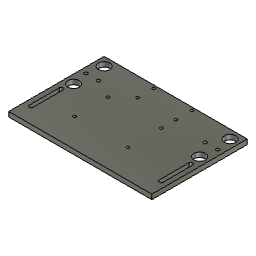
RollerPlate v14 (Autodesk Fusion 360 design; units mm, degrees)
Autodesk Fusion 360 part; units mm, degrees
sketch "Sketch1" plane through (0, 0, 0) normal (0, 0, 1) x (1, 0, 0)
  line L0 (-150, 100) -> (0, 100)
  line L1 (0, 100) -> (0, 0)
  line L2 (0, 0) -> (-150, 0)
  line L3 (-150, 0) -> (-150, 100)
  circle A0 centre (-135, 75) radius 3.25
  circle A1 centre (-115, 75) radius 3.25
  circle A2 centre (-35, 75) radius 3.25
  circle A3 centre (-15, 75) radius 3.25
  line L4 (-141, 48) -> (-141, 22)
  line L5 (-145, 22) -> (-145, 48)
  arc A4 (-143, 50) -> (-145, 48) centre (-143, 48) ccw
  arc A5 (-141, 48) -> (-143, 50) centre (-143, 48) ccw
  arc A6 (-145, 22) -> (-143, 20) centre (-143, 22) ccw
  arc A7 (-143, 20) -> (-141, 22) centre (-143, 22) ccw
  line L6 (-5, 48) -> (-5, 22)
  line L7 (-9, 22) -> (-9, 48)
  arc A8 (-7, 50) -> (-9, 48) centre (-7, 48) ccw
  arc A9 (-5, 48) -> (-7, 50) centre (-7, 48) ccw
  arc A10 (-9, 22) -> (-7, 20) centre (-7, 22) ccw
  arc A11 (-7, 20) -> (-5, 22) centre (-7, 22) ccw
  point P0 (-145, 50)
  point P1 (-141, 50)
  point P2 (-9, 50)
  point P3 (-5, 50)
  dimension "d1" = 150
  dimension "d2" = 100
  dimension "d3" = 6.5
  dimension "d4" = 25
  dimension "d5" = 15
  dimension "d6" = 6.5
  dimension "d7" = 6.5
  dimension "d8" = 6.5
  dimension "d9" = 20
  dimension "d10" = 15
  dimension "d11" = 20
  dimension "d53" = 4
  dimension "d55" = 5
  dimension "d57" = 2
  dimension "d58" = 2
  dimension "d59" = 2
  dimension "d60" = 4
  dimension "d62" = 5
  dimension "d64" = 2
  dimension "d65" = 2
  dimension "d66" = 2
  dimension "d67" = 2
  constraint horizontal L0
  constraint vertical L1
  constraint horizontal L2
  constraint vertical L3
  constraint coincident L1.end L2.start
  constraint vertical L4
  constraint vertical L5
  constraint coincident P0 L5
  constraint tangent L5 A4
  constraint coincident P1 L4
  constraint tangent L4 A5
  constraint coincident A4.start A5.end
  constraint tangent L5 A6
  constraint tangent L4 A7
  constraint equal A6 A7
  constraint coincident A6.end A7.start
  constraint vertical L6
  constraint vertical L7
  constraint coincident P2 L7
  constraint tangent L7 A8
  constraint coincident P3 L6
  constraint tangent L6 A9
  constraint coincident A8.start A9.end
  constraint tangent L7 A10
  constraint tangent L6 A11
  constraint coincident A10.end A11.start
  measures "d1" distance of L1 L3
  measures "d2" distance of L0 L2
  measures "d3" diameter of A0
  measures "d4" distance of L0 A0.centre
  measures "d5" distance of L3 A0.centre
  measures "d6" diameter of A1
  measures "d7" diameter of A2
  measures "d8" diameter of A3
  measures "d9" distance of A0.centre A1.centre
  measures "d10" distance of L1 A3.centre
  measures "d11" distance of A2.centre A3.centre
  measures "d53" distance of P0 P1
  measures "d55" distance of L3 L5
  measures "d57" radius of A4
  measures "d58" radius of A5
  measures "d59" radius of A6
  measures "d60" distance of P2 P3
  measures "d62" distance of L1 L6
  measures "d64" radius of A8
  measures "d65" radius of A9
  measures "d66" radius of A10
  measures "d67" radius of A11
extrude "Extrude1" add sketch "Sketch1" along normal blind 5 contours L0 L1 L2 L3 | L4 L5 A4 A5 A6 A7 | L6 L7 A8 A9 A10 A11 makes body 1
sketch "Sketch2" plane through (0, 0, 5) normal (0, 0, 1) x (-1, 0, 0)
  circle A0 centre (135, -75) radius 3.25
  circle A1 centre (35, -75) radius 3.25
  circle A2 centre (115, -75) radius 3.25
  circle A3 centre (15, -75) radius 3.25
  line L0 (150, 0) -> (0, 0)
  line L1 (0, 0) -> (0, -100)
  line L2 (0, -100) -> (150, -100)
  line L3 (150, -100) -> (150, 0)
  circle A4 centre (141, -91) radius 6
  circle A5 centre (141, -59) radius 6
  circle A6 centre (109, -91) radius 6
  circle A7 centre (109, -59) radius 6
  circle A8 centre (41, -91) radius 6
  circle A9 centre (41, -59) radius 6
  circle A10 centre (9, -91) radius 6
  circle A11 centre (9, -59) radius 6
  dimension "d25" = 12
  dimension "d26" = 9
  dimension "d27" = 9
  dimension "d28" = 12
  dimension "d29" = 12
  dimension "d30" = 12
  dimension "d31" = 12
  dimension "d32" = 12
  dimension "d33" = 12
  dimension "d34" = 12
  dimension "d35" = 9
  dimension "d36" = 9
  dimension "d37" = 41
  dimension "d38" = 41
  dimension "d39" = 41
  dimension "d40" = 41
  dimension "d41" = 9
  dimension "d42" = 9
  dimension "d43" = 41
  dimension "d44" = 41
  dimension "d45" = 9
  dimension "d46" = 9
  dimension "d47" = 41
  dimension "d48" = 41
  measures "d25" diameter of A4
  measures "d26" distance of L2 A4.centre
  measures "d27" distance of L3 A4.centre
  measures "d28" diameter of A5
  measures "d29" diameter of A6
  measures "d30" diameter of A7
  measures "d31" diameter of A8
  measures "d32" diameter of A9
  measures "d33" diameter of A10
  measures "d34" diameter of A11
  measures "d35" distance of L2 A6.centre
  measures "d36" distance of L3 A5.centre
  measures "d37" distance of L3 A6.centre
  measures "d38" distance of L3 A7.centre
  measures "d39" distance of L2 A5.centre
  measures "d40" distance of L2 A7.centre
  measures "d41" distance of L1 A10.centre
  measures "d42" distance of L1 A11.centre
  measures "d43" distance of L1 A8.centre
  measures "d44" distance of L1 A9.centre
  measures "d45" distance of L2 A10.centre
  measures "d46" distance of L2 A8.centre
  measures "d47" distance of L2 A11.centre
  measures "d48" distance of L2 A9.centre
extrude "Extrude2" cut sketch "Sketch2" against normal blind 5 contours A4 | A5 | A6 | A7 | A8 | A9 | A10 | A11 bodies 1
extrude "Extrude3" cut 1 faces at (-64.3973, 17.8049, 5) along direction (0, 0, -1) blind 1 on bodies 1 bodies 1
sketch "Sketch3" plane through (0, 0, 4) normal (0, 0, 1) x (-1, 0, 0)
  circle A0 centre (41, -91) radius 6
  circle A1 centre (141, -59) radius 6
  circle A2 centre (109, -59) radius 6
  circle A3 centre (9, -91) radius 6
  circle A4 centre (41, -59) radius 6
  circle A5 centre (141, -91) radius 6
  circle A6 centre (109, -91) radius 6
  circle A7 centre (9, -59) radius 6
  circle A8 centre (115, -75) radius 3.25
  circle A9 centre (135, -75) radius 3.25
  circle A10 centre (35, -75) radius 3.25
  circle A11 centre (15, -75) radius 3.25
  line L0 (150, 0) -> (0, 0)
  line L1 (0, 0) -> (0, -100)
  line L2 (0, -100) -> (150, -100)
  line L3 (150, -100) -> (150, 0)
  line L4 (144, -45) -> (142, -45)
  line L5 (141, -44) -> (141, -16)
  line L6 (142, -15) -> (144, -15)
  line L7 (145, -16) -> (145, -44)
  line L8 (8, -45) -> (6, -45)
  line L9 (5, -44) -> (5, -16)
  line L10 (6, -15) -> (8, -15)
  line L11 (9, -16) -> (9, -44)
  arc A12 (144, -45) -> (145, -44) centre (144, -44) ccw
  arc A13 (141, -44) -> (142, -45) centre (142, -44) ccw
  arc A14 (145, -16) -> (144, -15) centre (144, -16) ccw
  arc A15 (142, -15) -> (141, -16) centre (142, -16) ccw
  arc A16 (8, -45) -> (9, -44) centre (8, -44) ccw
  arc A17 (5, -44) -> (6, -45) centre (6, -44) ccw
  arc A18 (9, -16) -> (8, -15) centre (8, -16) ccw
  arc A19 (6, -15) -> (5, -16) centre (6, -16) ccw
  point P0 (145, -45)
  point P1 (141, -45)
  point P2 (9, -45)
  point P3 (5, -45)
  dimension "d70" = 4
  dimension "d71" = 30
  dimension "d72" = 55
  dimension "d73" = 5
  dimension "d74" = 4
  dimension "d75" = 30
  dimension "d76" = 55
  dimension "d77" = 5
  dimension "d78" = 1
  dimension "d79" = 1
  dimension "d80" = 1
  dimension "d81" = 1
  constraint horizontal L4
  constraint vertical L5
  constraint horizontal L6
  constraint vertical L7
  constraint horizontal L8
  constraint vertical L9
  constraint horizontal L10
  constraint vertical L11
  constraint coincident P0 L4
  constraint coincident P0 L7
  constraint tangent L4 A12
  constraint tangent L7 A12
  constraint coincident P1 L5
  constraint coincident P1 L4
  constraint tangent L5 A13
  constraint tangent L4 A13
  constraint tangent L7 A14
  constraint tangent L6 A14
  constraint equal A13 A14
  constraint tangent L5 A15
  constraint tangent L6 A15
  constraint equal A13 A15
  constraint coincident P2 L11
  constraint coincident P2 L8
  constraint tangent L11 A16
  constraint tangent L8 A16
  constraint coincident P3 L9
  constraint coincident P3 L8
  constraint tangent L9 A17
  constraint tangent L8 A17
  constraint tangent L10 A18
  constraint tangent L11 A18
  constraint equal A17 A18
  constraint tangent L9 A19
  constraint tangent L10 A19
  constraint equal A17 A19
  measures "d70" distance of P0 P1
  measures "d71" distance of L4 L6
  measures "d72" distance of L2 L4
  measures "d73" distance of L3 L7
  measures "d74" distance of P2 P3
  measures "d75" distance of L8 L10
  measures "d76" distance of L2 L8
  measures "d77" distance of L1 L9
  measures "d78" radius of A12
  measures "d79" radius of A13
  measures "d80" radius of A16
  measures "d81" radius of A17
extrude "Extrude5" cut sketch "Sketch3" against normal blind 5 contours L4 L5 L6 L7 A12 A13 A14 A15 | L8 L9 L10 L11 A16 A17 A18 A19 bodies 1
extrude "Extrude6" add 1 faces at (-64.6667, 28.3953, 4) along direction (0, 0, 1) blind 1 on bodies 1 bodies 1
extrude "Extrude7" cut 1 faces at (-64.6667, 28.3953, 5) along direction (0, 0, -1) blind 3 on bodies 1 bodies 1
extrude "Extrude8" add 1 faces at (-64.6667, 28.3953, 2) along direction (0, 0, 1) blind 3 on bodies 1 bodies 1
sketch "Sketch4" plane through (0, 0, 5) normal (0, 0, 1) x (-1, 0, 0)
  line L0 (142, -15) -> (144, -15)
  arc A0 (145, -16) -> (144, -15) centre (144, -16) ccw
  line L1 (145, -16) -> (145, -44)
  arc A1 (144, -45) -> (145, -44) centre (144, -44) ccw
  line L2 (144, -45) -> (142, -45)
  arc A2 (141, -44) -> (142, -45) centre (142, -44) ccw
  line L3 (141, -44) -> (141, -16)
  arc A3 (142, -15) -> (141, -16) centre (142, -16) ccw
  line L4 (6, -15) -> (8, -15)
  arc A4 (9, -16) -> (8, -15) centre (8, -16) ccw
  line L5 (9, -16) -> (9, -44)
  arc A5 (8, -45) -> (9, -44) centre (8, -44) ccw
  line L6 (8, -45) -> (6, -45)
  arc A6 (5, -44) -> (6, -45) centre (6, -44) ccw
  line L7 (5, -44) -> (5, -16)
  arc A7 (6, -15) -> (5, -16) centre (6, -16) ccw
  circle A8 centre (41, -91) radius 6
  circle A9 centre (141, -59) radius 6
  circle A10 centre (109, -59) radius 6
  circle A11 centre (9, -91) radius 6
  circle A12 centre (41, -59) radius 6
  circle A13 centre (141, -91) radius 6
  circle A14 centre (109, -91) radius 6
  circle A15 centre (9, -59) radius 6
  circle A16 centre (115, -75) radius 3.25
  circle A17 centre (135, -75) radius 3.25
  circle A18 centre (35, -75) radius 3.25
  circle A19 centre (15, -75) radius 3.25
  line L8 (150, 0) -> (0, 0)
  line L9 (0, 0) -> (0, -100)
  line L10 (0, -100) -> (150, -100)
  line L11 (150, -100) -> (150, 0)
  line L12 (75, -100) -> (75, 0)
  circle A20 centre (95, -34) radius 3.25
  circle A21 centre (55, -34) radius 3.25
  circle A22 centre (103, -75) radius 3.25
  circle A23 centre (95, -75) radius 3.25
  dimension "d96" = 6.5
  dimension "d97" = 20
  dimension "d99" = 6.5
  dimension "d100" = 20
  dimension "d102" = 34
  dimension "d103" = 34
  dimension "d104" = 6.5
  dimension "d105" = 6.5
  dimension "d106" = 28
  dimension "d108" = 25
  dimension "d109" = 25
  dimension "d113" = 20
  constraint midpoint L10 L12.start
  constraint midpoint L8 L12.end
  measures "d96" diameter of A20
  measures "d97" distance of L12 A20.centre
  measures "d99" diameter of A21
  measures "d100" distance of L12 A21.centre
  measures "d102" distance of L8 A20.centre
  measures "d103" distance of L8 A21.centre
  measures "d104" diameter of A22
  measures "d105" diameter of A23
  measures "d106" distance of L12 A22.centre
  measures "d108" distance of L10 A22.centre
  measures "d109" distance of L10 A23.centre
  measures "d113" distance of L12 A23.centre
extrude "Extrude9" cut sketch "Sketch4" against normal blind 8 contours A20 | A21 | A22 | A23 bodies 1
sketch "Sketch5" plane through (0, 0, 0) normal (0, 0, 1) x (1, 0, 0)
  circle A0 centre (-103, 75) radius 3.25
  circle A1 centre (-95, 75) radius 3.25
  dimension "d116" = 6.5
  dimension "d117" = 6.5
  measures "d116" diameter of A0
  measures "d117" diameter of A1
extrude "Extrude10" add sketch "Sketch5" along normal blind 5 bodies 1
sketch "Sketch6" plane through (0, 0, 5) normal (0, 0, 1) x (-1, 0, 0)
  circle A0 centre (95, -34) radius 3.25
  circle A1 centre (55, -34) radius 3.25
  line L0 (142, -15) -> (144, -15)
  arc A2 (145, -16) -> (144, -15) centre (144, -16) ccw
  line L1 (145, -16) -> (145, -44)
  arc A3 (144, -45) -> (145, -44) centre (144, -44) ccw
  line L2 (144, -45) -> (142, -45)
  arc A4 (141, -44) -> (142, -45) centre (142, -44) ccw
  line L3 (141, -44) -> (141, -16)
  arc A5 (142, -15) -> (141, -16) centre (142, -16) ccw
  line L4 (6, -15) -> (8, -15)
  arc A6 (9, -16) -> (8, -15) centre (8, -16) ccw
  line L5 (9, -16) -> (9, -44)
  arc A7 (8, -45) -> (9, -44) centre (8, -44) ccw
  line L6 (8, -45) -> (6, -45)
  arc A8 (5, -44) -> (6, -45) centre (6, -44) ccw
  line L7 (5, -44) -> (5, -16)
  arc A9 (6, -15) -> (5, -16) centre (6, -16) ccw
  circle A10 centre (41, -91) radius 6
  circle A11 centre (141, -59) radius 6
  circle A12 centre (109, -59) radius 6
  circle A13 centre (9, -91) radius 6
  circle A14 centre (41, -59) radius 6
  circle A15 centre (141, -91) radius 6
  circle A16 centre (109, -91) radius 6
  circle A17 centre (9, -59) radius 6
  circle A18 centre (115, -75) radius 3.25
  circle A19 centre (135, -75) radius 3.25
  circle A20 centre (35, -75) radius 3.25
  circle A21 centre (15, -75) radius 3.25
  line L8 (150, 0) -> (0, 0)
  line L9 (0, 0) -> (0, -100)
  line L10 (0, -100) -> (150, -100)
  line L11 (150, -100) -> (150, 0)
  circle A22 centre (75, -90) radius 3
  circle A23 centre (75, -60) radius 3
  circle A24 centre (94, -90) radius 1.5
  circle A25 centre (94, -60) radius 1.5
  circle A26 centre (56, -90) radius 1.5
  circle A27 centre (56, -60) radius 1.5
  dimension "d120" = 6
  dimension "d121" = 6
  dimension "d122" = 3
  dimension "d123" = 3
  dimension "d124" = 3
  dimension "d125" = 3
  dimension "d126" = 75
  dimension "d127" = 75
  dimension "d128" = 19
  dimension "d129" = 19
  dimension "d130" = 19
  dimension "d131" = 19
  dimension "d132" = 10
  dimension "d133" = 10
  dimension "d134" = 40
  dimension "d135" = 40
  dimension "d136" = 40
  dimension "d137" = 10
  measures "d120" diameter of A22
  measures "d121" diameter of A23
  measures "d122" diameter of A24
  measures "d123" diameter of A25
  measures "d124" diameter of A26
  measures "d125" diameter of A27
  measures "d126" distance of L11 A22.centre
  measures "d127" distance of L11 A23.centre
  measures "d128" horizontal distance of A22.centre A24.centre
  measures "d129" horizontal distance of A22.centre A26.centre
  measures "d130" horizontal distance of A23.centre A25.centre
  measures "d131" horizontal distance of A23.centre A27.centre
  measures "d132" distance of L10 A24.centre
  measures "d133" distance of L10 A26.centre
  measures "d134" distance of L10 A25.centre
  measures "d135" distance of L10 A27.centre
  measures "d136" distance of L10 A23.centre
  measures "d137" distance of L10 A22.centre
extrude "Extrude11" cut sketch "Sketch6" against normal blind 5 contours A22 | A23 | A24 | A25 | A26 | A27 bodies 1
sketch "Sketch7" plane through (0, 0, 5) normal (0, 0, 1) x (-1, 0, 0)
  circle A0 centre (75, -60) radius 3
  circle A1 centre (94, -90) radius 1.5
  circle A2 centre (56, -90) radius 1.5
  circle A3 centre (94, -60) radius 1.5
  circle A4 centre (75, -90) radius 3
  circle A5 centre (56, -60) radius 1.5
  circle A6 centre (95, -34) radius 3.25
  circle A7 centre (55, -34) radius 3.25
  line L0 (142, -15) -> (144, -15)
  arc A8 (145, -16) -> (144, -15) centre (144, -16) ccw
  line L1 (145, -16) -> (145, -44)
  arc A9 (144, -45) -> (145, -44) centre (144, -44) ccw
  line L2 (144, -45) -> (142, -45)
  arc A10 (141, -44) -> (142, -45) centre (142, -44) ccw
  line L3 (141, -44) -> (141, -16)
  arc A11 (142, -15) -> (141, -16) centre (142, -16) ccw
  line L4 (6, -15) -> (8, -15)
  arc A12 (9, -16) -> (8, -15) centre (8, -16) ccw
  line L5 (9, -16) -> (9, -44)
  arc A13 (8, -45) -> (9, -44) centre (8, -44) ccw
  line L6 (8, -45) -> (6, -45)
  arc A14 (5, -44) -> (6, -45) centre (6, -44) ccw
  line L7 (5, -44) -> (5, -16)
  arc A15 (6, -15) -> (5, -16) centre (6, -16) ccw
  circle A16 centre (41, -91) radius 6
  circle A17 centre (141, -59) radius 6
  circle A18 centre (109, -59) radius 6
  circle A19 centre (9, -91) radius 6
  circle A20 centre (41, -59) radius 6
  circle A21 centre (141, -91) radius 6
  circle A22 centre (109, -91) radius 6
  circle A23 centre (9, -59) radius 6
  circle A24 centre (115, -75) radius 3.25
  circle A25 centre (135, -75) radius 3.25
  circle A26 centre (35, -75) radius 3.25
  circle A27 centre (15, -75) radius 3.25
  line L8 (150, 0) -> (0, 0)
  line L9 (0, 0) -> (0, -100)
  line L10 (0, -100) -> (150, -100)
  line L11 (150, -100) -> (150, 0)
sketch "Sketch8" plane through (0, 0, 0) normal (0, 0, 1) x (1, 0, 0)
  circle A0 centre (-95, 34) radius 3.25
  circle A1 centre (-55, 34) radius 3.25
  dimension "d140" = 6.5
  dimension "d141" = 6.5
  measures "d140" diameter of A0
  measures "d141" diameter of A1
extrude "Extrude12" add sketch "Sketch8" along normal blind 5 bodies 1
sketch "Sketch9" plane through (0, 0, 5) normal (0, 0, 1) x (1, 0, 0)
  circle A0 centre (-94, 50) radius 1.5
  circle A1 centre (-94, 10) radius 1.5
  line L0 (-150, 100) -> (-150, 0)
  dimension "d144" = 3
  dimension "d145" = 3
  dimension "d164" = 56
  dimension "d165" = 56
  measures "d144" diameter of A0
  measures "d145" diameter of A1
  measures "d164" distance of A0.centre L0
  measures "d165" distance of A1.centre L0
extrude "Extrude13" cut sketch "Sketch9" against normal blind 5 bodies 1
sketch "Sketch10" plane through (0, 0, 5) normal (0, 0, 1) x (1, 0, 0)
  circle A0 centre (-144, 75) radius 1.75
  line L0 (0, 100) -> (-150, 100)
  line L1 (-150, 100) -> (-150, 0)
  circle A1 centre (-6, 75) radius 1.75
  line L2 (0, 0) -> (0, 100)
  dimension "d148" = 3.5
  dimension "d149" = 25
  dimension "d150" = 6
  dimension "d151" = 3.5
  dimension "d152" = 25
  dimension "d153" = 6
  measures "d148" diameter of A0
  measures "d149" distance of A0.centre L0
  measures "d150" distance of A0.centre L1
  measures "d151" diameter of A1
  measures "d152" distance of L0 A1.centre
  measures "d153" distance of A1.centre L2
extrude "Extrude14" cut sketch "Sketch10" against normal blind 6 bodies 1
sketch "Sketch11" plane through (0, 0, 5) normal (0, 0, 1) x (1, 0, 0)
  circle A0 centre (-56, 50) radius 1.5
  line L0 (0, 100) -> (-150, 100)
  line L1 (0, 0) -> (0, 100)
  circle A1 centre (-56, 10) radius 1.5
  dimension "d156" = 3
  dimension "d157" = 50
  dimension "d158" = 56
  dimension "d159" = 3
  dimension "d160" = 56
  dimension "d161" = 90
  measures "d156" diameter of A0
  measures "d157" distance of A0.centre L0
  measures "d158" distance of A0.centre L1
  measures "d159" diameter of A1
  measures "d160" distance of L1 A1.centre
  measures "d161" distance of L0 A1.centre
extrude "Extrude15" cut sketch "Sketch11" against normal blind 5 bodies 1
extrude "Extrude4" cut sketch "Sketch1" along normal blind 50 contours L4 L5 A4 A5 A6 A7 | L6 L7 A8 A9 A10 A11 bodies 1
sketch "Sketch12" plane through (0, 0, 5) normal (0, 0, 1) x (1, 0, 0)
  circle A0 centre (-56, 60) radius 1.4142
  circle A1 centre (-56, 50) radius 1.4142
  circle A2 centre (-94, 50) radius 1.4142
  circle A3 centre (-94, 60) radius 1.4142
  circle A4 centre (-94, 90) radius 1.4142
  circle A5 centre (-56, 90) radius 1.4142
  circle A6 centre (-75, 90) radius 3
  circle A7 centre (-75, 60) radius 3
  circle A8 centre (-135, 75) radius 3.25
  circle A9 centre (-115, 75) radius 3.25
  circle A10 centre (-109, 91) radius 6
  circle A11 centre (-109, 59) radius 6
  circle A12 centre (-35, 75) radius 3.25
  circle A13 centre (-41, 91) radius 6
  circle A14 centre (-15, 75) radius 3.25
  circle A15 centre (-41, 59) radius 6
  circle A16 centre (-94, 10) radius 1.5
  circle A17 centre (-56, 10) radius 1.5
  dimension "d166" = 6.5
  dimension "d167" = 6.5
  dimension "d168" = 12
  dimension "d169" = 12
  dimension "d170" = 6.5
  dimension "d171" = 12
  dimension "d172" = 6.5
  dimension "d173" = 12
  dimension "d174" = 3
  dimension "d175" = 3
  measures "d166" diameter of A8
  measures "d167" diameter of A9
  measures "d168" diameter of A10
  measures "d169" diameter of A11
  measures "d170" diameter of A12
  measures "d171" diameter of A13
  measures "d172" diameter of A14
  measures "d173" diameter of A15
  measures "d174" diameter of A16
  measures "d175" diameter of A17
extrude "Extrude16" add sketch "Sketch12" sketch "Sketch7" against normal blind 5 contours A1 | A2 | A8 | A16 | A17 of sketch 2 contours A0 | A1 | A2 | A3 | A4 | A5 | A16 | A18 | A20 | A22 | A24 | A26 | A27 bodies 1 makes body 2 at (-56.8255, 48.8517, 1.6667) makes body 3 at (-92.6711, 50.4837, 1.6667)
sketch "Sketch13" plane through (0, 0, 5) normal (0, 0, 1) x (-1, 0, 0)
  line L0 (5, -48) -> (5, -16)
  arc A0 (6, -15) -> (5, -16) centre (6, -16) ccw
  line L1 (6, -15) -> (8, -15)
  arc A1 (9, -16) -> (8, -15) centre (8, -16) ccw
  line L2 (9, -16) -> (9, -48)
  arc A2 (5, -48) -> (9, -48) centre (7, -48) ccw
  line L3 (141, -48) -> (141, -16)
  arc A3 (142, -15) -> (141, -16) centre (142, -16) ccw
  line L4 (142, -15) -> (144, -15)
  arc A4 (145, -16) -> (144, -15) centre (144, -16) ccw
  line L5 (145, -16) -> (145, -48)
  arc A5 (141, -48) -> (145, -48) centre (143, -48) ccw
  circle A6 centre (56, -50) radius 1.5
  circle A7 centre (144, -75) radius 1.75
  circle A8 centre (6, -75) radius 1.75
  circle A9 centre (94, -50) radius 1.5
  circle A10 centre (141, -59) radius 6
  circle A11 centre (9, -91) radius 6
  circle A12 centre (141, -91) radius 6
  circle A13 centre (9, -59) radius 6
  line L6 (150, 0) -> (0, 0)
  line L7 (0, 0) -> (0, -100)
  line L8 (0, -100) -> (150, -100)
  line L9 (150, -100) -> (150, 0)
  circle A14 centre (131, -75) radius 1.75
  circle A15 centre (19, -75) radius 1.75
  dimension "d178" = 3.5
  dimension "d179" = 13
  dimension "d180" = 3.5
  dimension "d181" = 13
  measures "d178" diameter of A14
  measures "d179" distance of A7.centre A14.centre
  measures "d180" diameter of A15
  measures "d181" distance of A8.centre A15.centre
extrude "Extrude17" cut sketch "Sketch13" against normal blind 8 contours A14 | A15 bodies 1
sketch "Sketch14" plane through (0, 0, 5) normal (0, 0, 1) x (-1, 0, 0)
  circle A0 centre (19, -75) radius 1.75
  circle A1 centre (131, -75) radius 1.75
  line L0 (5, -48) -> (5, -16)
  arc A2 (6, -15) -> (5, -16) centre (6, -16) ccw
  line L1 (6, -15) -> (8, -15)
  arc A3 (9, -16) -> (8, -15) centre (8, -16) ccw
  line L2 (9, -16) -> (9, -48)
  arc A4 (5, -48) -> (9, -48) centre (7, -48) ccw
  line L3 (141, -48) -> (141, -16)
  arc A5 (142, -15) -> (141, -16) centre (142, -16) ccw
  line L4 (142, -15) -> (144, -15)
  arc A6 (145, -16) -> (144, -15) centre (144, -16) ccw
  line L5 (145, -16) -> (145, -48)
  arc A7 (141, -48) -> (145, -48) centre (143, -48) ccw
  circle A8 centre (56, -50) radius 1.5
  circle A9 centre (144, -75) radius 1.75
  circle A10 centre (6, -75) radius 1.75
  circle A11 centre (94, -50) radius 1.5
  circle A12 centre (141, -59) radius 6
  circle A13 centre (9, -91) radius 6
  circle A14 centre (141, -91) radius 6
  circle A15 centre (9, -59) radius 6
  line L6 (150, 0) -> (0, 0)
  line L7 (0, 0) -> (0, -100)
  line L8 (0, -100) -> (150, -100)
  line L9 (150, -100) -> (150, 0)
  line L10 (75, -100) -> (75, -25) construction
  circle A16 centre (95, -97) radius 1.5
  circle A17 centre (95, -80) radius 1.5
  circle A18 centre (55, -97) radius 1.5
  circle A19 centre (55, -80) radius 1.5
  dimension "d184" = 3
  dimension "d185" = 3
  dimension "d186" = 3
  dimension "d187" = 3
  dimension "d188" = 3
  dimension "d189" = 3
  dimension "d190" = 20
  dimension "d191" = 20
  constraint midpoint L8 L10.start
  constraint perpendicular L8 L10
  measures "d184" diameter of A16
  measures "d185" diameter of A17
  measures "d186" diameter of A18
  measures "d187" diameter of A19
  measures "d188" distance of L8 A16.centre
  measures "d189" distance of L8 A18.centre
  measures "d190" distance of L8 A17.centre
  measures "d191" distance of L8 A19.centre
extrude "Extrude18" cut sketch "Sketch14" against normal blind 10 contours A16 | A17 | A18 | A19 bodies 1
sketch "Sketch15" plane through (0, 0, 5) normal (0, 0, 1) x (-1, 0, 0)
  circle A0 centre (95, -80) radius 1.5
  circle A1 centre (55, -80) radius 1.5
  circle A2 centre (95, -97) radius 1.5
  circle A3 centre (55, -97) radius 1.5
  circle A4 centre (19, -75) radius 1.75
  circle A5 centre (131, -75) radius 1.75
  line L0 (5, -48) -> (5, -16)
  arc A6 (6, -15) -> (5, -16) centre (6, -16) ccw
  line L1 (6, -15) -> (8, -15)
  arc A7 (9, -16) -> (8, -15) centre (8, -16) ccw
  line L2 (9, -16) -> (9, -48)
  arc A8 (5, -48) -> (9, -48) centre (7, -48) ccw
  line L3 (141, -48) -> (141, -16)
  arc A9 (142, -15) -> (141, -16) centre (142, -16) ccw
  line L4 (142, -15) -> (144, -15)
  arc A10 (145, -16) -> (144, -15) centre (144, -16) ccw
  line L5 (145, -16) -> (145, -48)
  arc A11 (141, -48) -> (145, -48) centre (143, -48) ccw
  circle A12 centre (144, -75) radius 1.75
  circle A13 centre (6, -75) radius 1.75
  circle A14 centre (141, -59) radius 6
  circle A15 centre (9, -91) radius 6
  circle A16 centre (141, -91) radius 6
  circle A17 centre (9, -59) radius 6
  line L6 (150, 0) -> (0, 0)
  line L7 (0, 0) -> (0, -100)
  line L8 (0, -100) -> (150, -100)
  line L9 (150, -100) -> (150, 0)
  circle A18 centre (92.5, -55) radius 1.5
  circle A19 centre (92.5, -2.5) radius 1.5
  circle A20 centre (57.5, -55) radius 1.5
  circle A21 centre (57.5, -2.5) radius 1.5
  line L10 (75, -100) -> (75, 0) construction
  line L11 (150, -50) -> (0, -50) construction
  dimension "d194" = 3
  dimension "d195" = 3
  dimension "d196" = 3
  dimension "d197" = 3
  dimension "d198" = 17.5
  dimension "d199" = 17.5
  dimension "d200" = 17.5
  dimension "d201" = 17.5
  dimension "d203" = 52.5
  dimension "d204" = 45
  dimension "d205" = 45
  dimension "d206" = 52.5
  constraint midpoint L8 L10.start
  constraint midpoint L6 L10.end
  constraint midpoint L9 L11.start
  constraint midpoint L7 L11.end
  measures "d194" diameter of A18
  measures "d195" diameter of A19
  measures "d196" diameter of A20
  measures "d197" diameter of A21
  measures "d198" distance of A18.centre L10
  measures "d199" distance of A19.centre L10
  measures "d200" distance of A20.centre L10
  measures "d201" distance of A21.centre L10
  measures "d203" distance of A18.centre A19.centre
  measures "d204" distance of L8 A18.centre
  measures "d205" distance of L8 A20.centre
  measures "d206" distance of A20.centre A21.centre
extrude "Extrude19" cut sketch "Sketch15" against normal blind 10 contours A18 | A19 | A20 | A21 bodies 1
sketch "Sketch16" plane through (0, 0, 5) normal (0, 0, 1) x (-1, 0, 0)
  circle A0 centre (57.5, -55) radius 1.5
  circle A1 centre (92.5, -2.5) radius 1.5
  circle A2 centre (92.5, -55) radius 1.5
  circle A3 centre (57.5, -2.5) radius 1.5
  circle A4 centre (95, -80) radius 1.5
  circle A5 centre (55, -80) radius 1.5
  circle A6 centre (95, -97) radius 1.5
  circle A7 centre (55, -97) radius 1.5
  circle A8 centre (19, -75) radius 1.75
  circle A9 centre (131, -75) radius 1.75
  line L0 (5, -48) -> (5, -16)
  arc A10 (6, -15) -> (5, -16) centre (6, -16) ccw
  line L1 (6, -15) -> (8, -15)
  arc A11 (9, -16) -> (8, -15) centre (8, -16) ccw
  line L2 (9, -16) -> (9, -48)
  arc A12 (5, -48) -> (9, -48) centre (7, -48) ccw
  line L3 (141, -48) -> (141, -16)
  arc A13 (142, -15) -> (141, -16) centre (142, -16) ccw
  line L4 (142, -15) -> (144, -15)
  arc A14 (145, -16) -> (144, -15) centre (144, -16) ccw
  line L5 (145, -16) -> (145, -48)
  arc A15 (141, -48) -> (145, -48) centre (143, -48) ccw
  circle A16 centre (56, -50) radius 1.5
  circle A17 centre (144, -75) radius 1.75
  circle A18 centre (6, -75) radius 1.75
  circle A19 centre (94, -50) radius 1.5
  circle A20 centre (141, -59) radius 6
  circle A21 centre (9, -91) radius 6
  circle A22 centre (141, -91) radius 6
  circle A23 centre (9, -59) radius 6
  line L6 (150, 0) -> (0, 0)
  line L7 (0, 0) -> (0, -100)
  line L8 (0, -100) -> (150, -100)
  line L9 (150, -100) -> (150, 0)
  circle A24 centre (92.5, -55) radius 1.5
  circle A25 centre (94, -50) radius 1.5
  circle A26 centre (57.5, -55) radius 1.5
  circle A27 centre (57.5, -2.5) radius 1.5
  circle A28 centre (92.5, -2.5) radius 1.5
  dimension "d209" = 3
  dimension "d210" = 3
  dimension "d211" = 3
  constraint concentric A2 A24
  constraint concentric A19 A25
  constraint concentric A0 A26
  constraint concentric A3 A27
  constraint concentric A1 A28
  measures "d209" diameter of A24
  measures "d210" diameter of A27
  measures "d211" diameter of A28
extrude "Extrude20" cut sketch "Sketch16" against normal blind 5 contours A0 A26 | A1 A28 | A2 A24 | A3 A27 | A16 | A19 A25 bodies 2 3
sketch "Sketch17" plane through (0, 0, 5) normal (0, 0, 1) x (-1, 0, 0)
  circle A0 centre (57.5, -55) radius 1.5
  circle A1 centre (92.5, -2.5) radius 1.5
  circle A2 centre (92.5, -55) radius 1.5
  circle A3 centre (57.5, -2.5) radius 1.5
  circle A4 centre (95, -80) radius 1.5
  circle A5 centre (55, -80) radius 1.5
  circle A6 centre (95, -97) radius 1.5
  circle A7 centre (55, -97) radius 1.5
  circle A8 centre (19, -75) radius 1.75
  circle A9 centre (131, -75) radius 1.75
  line L0 (5, -48) -> (5, -16)
  arc A10 (6, -15) -> (5, -16) centre (6, -16) ccw
  line L1 (6, -15) -> (8, -15)
  arc A11 (9, -16) -> (8, -15) centre (8, -16) ccw
  line L2 (9, -16) -> (9, -48)
  arc A12 (5, -48) -> (9, -48) centre (7, -48) ccw
  line L3 (141, -48) -> (141, -16)
  arc A13 (142, -15) -> (141, -16) centre (142, -16) ccw
  line L4 (142, -15) -> (144, -15)
  arc A14 (145, -16) -> (144, -15) centre (144, -16) ccw
  line L5 (145, -16) -> (145, -48)
  arc A15 (141, -48) -> (145, -48) centre (143, -48) ccw
  circle A16 centre (56, -50) radius 1.5
  circle A17 centre (144, -75) radius 1.75
  circle A18 centre (6, -75) radius 1.75
  circle A19 centre (94, -50) radius 1.5
  circle A20 centre (141, -59) radius 6
  circle A21 centre (9, -91) radius 6
  circle A22 centre (141, -91) radius 6
  circle A23 centre (9, -59) radius 6
  line L6 (150, 0) -> (0, 0)
  line L7 (0, 0) -> (0, -100)
  line L8 (0, -100) -> (150, -100)
  line L9 (150, -100) -> (150, 0)
  circle A24 centre (57.5, -2.5) radius 1.5
  circle A25 centre (92.5, -2.5) radius 1.5
  circle A26 centre (94, -50) radius 1.5
  circle A27 centre (92.5, -55) radius 1.5
  circle A28 centre (57.5, -55) radius 1.5
  circle A29 centre (56, -50) radius 1.5
  dimension "d214" = 3
  dimension "d215" = 3
  dimension "d216" = 3
  dimension "d217" = 3
  dimension "d218" = 3
  dimension "d219" = 3
  constraint concentric A3 A24
  constraint concentric A1 A25
  constraint concentric A19 A26
  constraint concentric A2 A27
  constraint concentric A0 A28
  constraint concentric A16 A29
  measures "d214" diameter of A24
  measures "d215" diameter of A25
  measures "d216" diameter of A26
  measures "d217" diameter of A27
  measures "d218" diameter of A28
  measures "d219" diameter of A29
extrude "Extrude21" add sketch "Sketch17" against normal blind 5 contours A0 A28 | A1 A25 | A2 A27 | A3 A24 | A16 A29 | A19 A26 bodies 1 2 3
sketch "Sketch18" plane through (0, 0, 5) normal (0, 0, 1) x (-1, 0, 0)
  circle A0 centre (95, -80) radius 1.5
  circle A1 centre (55, -80) radius 1.5
  circle A2 centre (95, -97) radius 1.5
  circle A3 centre (55, -97) radius 1.5
  circle A4 centre (19, -75) radius 1.75
  circle A5 centre (131, -75) radius 1.75
  line L0 (5, -48) -> (5, -16)
  arc A6 (6, -15) -> (5, -16) centre (6, -16) ccw
  line L1 (6, -15) -> (8, -15)
  arc A7 (9, -16) -> (8, -15) centre (8, -16) ccw
  line L2 (9, -16) -> (9, -48)
  arc A8 (5, -48) -> (9, -48) centre (7, -48) ccw
  line L3 (141, -48) -> (141, -16)
  arc A9 (142, -15) -> (141, -16) centre (142, -16) ccw
  line L4 (142, -15) -> (144, -15)
  arc A10 (145, -16) -> (144, -15) centre (144, -16) ccw
  line L5 (145, -16) -> (145, -48)
  arc A11 (141, -48) -> (145, -48) centre (143, -48) ccw
  circle A12 centre (144, -75) radius 1.75
  circle A13 centre (6, -75) radius 1.75
  circle A14 centre (141, -59) radius 6
  circle A15 centre (9, -91) radius 6
  circle A16 centre (141, -91) radius 6
  circle A17 centre (9, -59) radius 6
  line L6 (150, 0) -> (0, 0)
  line L7 (0, 0) -> (0, -100)
  line L8 (0, -100) -> (150, -100)
  line L9 (150, -100) -> (150, 0)
  circle A18 centre (55, -65) radius 1.5
  circle A19 centre (55, -30) radius 1.5
  circle A20 centre (111, -65) radius 1.5
  circle A21 centre (111, -30) radius 1.5
  dimension "d222" = 3
  dimension "d223" = 3
  dimension "d224" = 35
  dimension "d225" = 3
  dimension "d226" = 56
  dimension "d227" = 3
  dimension "d228" = 56
  measures "d222" diameter of A18
  measures "d223" diameter of A19
  measures "d224" distance of A18.centre A19.centre
  measures "d225" diameter of A20
  measures "d226" distance of A18.centre A20.centre
  measures "d227" diameter of A21
  measures "d228" distance of A19.centre A21.centre
extrude "Extrude22" cut sketch "Sketch18" against normal blind 5 contours A18 | A19 | A20 | A21 bodies 1
sketch "Sketch19" plane through (0, 0, 5) normal (0, 0, 1) x (-1, 0, 0)
  circle A0 centre (55, -65) radius 1.5
  circle A1 centre (111, -65) radius 1.5
  circle A2 centre (55, -30) radius 1.5
  circle A3 centre (111, -30) radius 1.5
  circle A4 centre (95, -80) radius 1.5
  circle A5 centre (55, -80) radius 1.5
  circle A6 centre (95, -97) radius 1.5
  circle A7 centre (55, -97) radius 1.5
  circle A8 centre (19, -75) radius 1.75
  circle A9 centre (131, -75) radius 1.75
  line L0 (5, -48) -> (5, -16)
  arc A10 (6, -15) -> (5, -16) centre (6, -16) ccw
  line L1 (6, -15) -> (8, -15)
  arc A11 (9, -16) -> (8, -15) centre (8, -16) ccw
  line L2 (9, -16) -> (9, -48)
  arc A12 (5, -48) -> (9, -48) centre (7, -48) ccw
  line L3 (141, -48) -> (141, -16)
  arc A13 (142, -15) -> (141, -16) centre (142, -16) ccw
  line L4 (142, -15) -> (144, -15)
  arc A14 (145, -16) -> (144, -15) centre (144, -16) ccw
  line L5 (145, -16) -> (145, -48)
  arc A15 (141, -48) -> (145, -48) centre (143, -48) ccw
  circle A16 centre (144, -75) radius 1.75
  circle A17 centre (6, -75) radius 1.75
  circle A18 centre (141, -59) radius 6
  circle A19 centre (9, -91) radius 6
  circle A20 centre (141, -91) radius 6
  circle A21 centre (9, -59) radius 6
  line L6 (150, 0) -> (0, 0)
  line L7 (0, 0) -> (0, -100)
  line L8 (0, -100) -> (150, -100)
  line L9 (150, -100) -> (150, 0)
sketch "Sketch20" plane through (0, 0, 5) normal (0, 0, 1) x (1, 0, 0)
